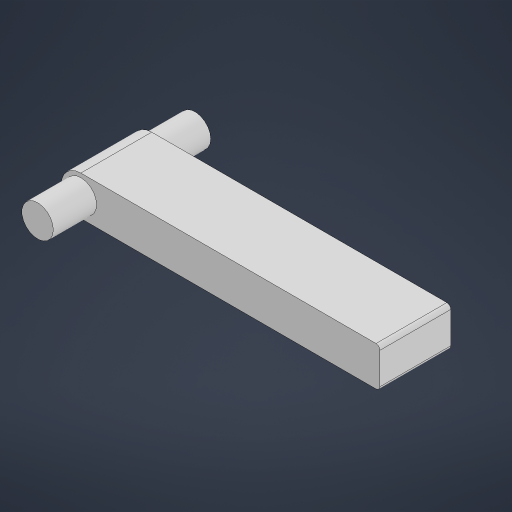
# Autodesk Inventor part: 집게 고정
Saved by Autodesk Inventor 2024 (Build 280153000, 153)
## iProperties
Created: 2024-01-27
Part Number: 집게 고정
Material: 일반
Document SubType Name: Modeling
Designer: likek
Density: 1 g/cm^3
Appearance: 기본값
Author: likek
Autodesk Inventor part; units mm, degrees
ref_plane "YZ Plane" through (0, 0, 0) normal (1, 0, 0) x (0, 1, 0)
ref_plane "XZ Plane" through (0, 0, 0) normal (0, 1, 0) x (-1, 0, 0)
ref_plane "XY Plane" through (0, 0, 0) normal (0, 0, 1) x (1, 0, 0)
sketch "스케치1" plane through (0, 0, 0) normal (0, 0, 1) x (1, 0, 0)
  circle A0 centre (0, 0) radius 0.4
  circle A1 centre (0, 0) radius 0.5
  line L0 (0, 0.5) -> (7.6, 0.5)
  line L1 (7.6, 0.5) -> (7.6, -0.5)
  line L2 (7.6, -0.5) -> (0, -0.5)
  line L3 (0, -0.5) -> (0, 0.5)
  point P0 (0, -0.5)
  dimension "d1" = 1
  dimension "d0" = 0.8
  dimension "d2" = 1
  dimension "d7" = 7.6
  constraints: 8 end point, 2 coincident, 2 parallel, 1 centre point, 1 horizontal, 1 perpendicular, 3 other
  measures "d0" diameter of A0
  measures "d2" distance of L0.end L1.end
  measures "d7" distance of L0.start L0.end
extrude "돌출1" add sketch "스케치1" along normal mid plane 4 contours A0 L3 | L3 A0
extrude "돌출2" add sketch "스케치1" along normal mid plane 1.8 contours A0 L3 A1 | A0 L3 A1 | L0 L1 L2 A1
fillet "모깎기1" radius 0.1 2 edges at (7.6, 0.5, 0) (7.6, -0.5, 0)
